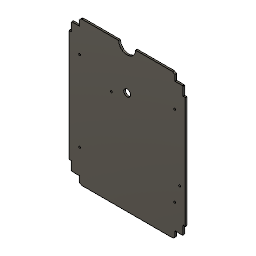
baseplate v1_wire_hole (Autodesk Fusion 360 design; units mm, degrees)
Autodesk Fusion 360 part; units mm, degrees
sketch "Sketch1" plane through (0, 0, 0) normal (0, 0, 1) x (1, 0, 0)
  line L0 (100, 125) -> (-100, 125)
  line L1 (-100, 125) -> (-100, -125)
  line L2 (-100, -125) -> (100, -125)
  line L3 (100, -125) -> (100, 125)
  line L4 (100, 125) -> (-100, -125) construction
  line L5 (-100, 125) -> (100, -125) construction
  line L6 (-100, 125) -> (100, 125)
  line L7 (100, 125) -> (100, 129)
  line L8 (100, 129) -> (-100, 129)
  line L9 (-100, 129) -> (-100, 125)
  line L10 (-100, -125) -> (100, -125)
  line L11 (100, -125) -> (100, -129)
  line L12 (100, -129) -> (-100, -129)
  line L13 (-100, -129) -> (-100, -125)
  line L14 (100, 125) -> (104, 125)
  line L15 (104, 125) -> (104, -125)
  line L16 (104, -125) -> (100, -125)
  line L17 (100, -125) -> (100, 125)
  line L18 (-100, 125) -> (-104, 125)
  line L19 (-104, 125) -> (-104, -125)
  line L20 (-104, -125) -> (-100, -125)
  line L21 (-100, -125) -> (-100, 125)
  line L22 (-80, -53.8) -> (-80, 2.2) construction
  circle A0 centre (-80, -53.8) radius 1.65 construction
  circle A1 centre (-80, 2.2) radius 1.65 construction
  line L23 (-61.0622, -1) -> (-98.9378, -1) construction
  line L24 (-98.9378, -1) -> (-98.9378, -50.6) construction
  line L25 (-98.9378, -50.6) -> (-61.0622, -50.6) construction
  line L26 (-61.0622, -50.6) -> (-61.0622, -1) construction
  line L27 (-61.0622, -1) -> (-98.9378, -50.6) construction
  line L28 (-98.9378, -1) -> (-61.0622, -50.6) construction
  line L29 (-30.5, 49.5) -> (98.5, 49.5) construction
  line L30 (98.5, 49.5) -> (98.5, -47.5) construction
  line L31 (98.5, -47.5) -> (-30.5, -47.5) construction
  line L32 (-30.5, -47.5) -> (-30.5, 49.5) construction
  circle A2 centre (-28, 43) radius 1.65
  circle A3 centre (94, -42) radius 1.65
  line L33 (-100, 125) -> (-85.5, 125)
  line L34 (-85.5, 125) -> (-85.5, 116)
  line L35 (-85.5, 116) -> (-100, 116)
  line L36 (-100, 116) -> (-100, 125)
  line L37 (100, 125) -> (85.5, 125)
  line L38 (85.5, 125) -> (85.5, 116)
  line L39 (85.5, 116) -> (100, 116)
  line L40 (100, 116) -> (100, 125)
  line L41 (-100, -125) -> (-85.5, -125)
  line L42 (-85.5, -125) -> (-85.5, -116)
  line L43 (-85.5, -116) -> (-100, -116)
  line L44 (-100, -116) -> (-100, -125)
  line L45 (100, -125) -> (85.5, -125)
  line L46 (85.5, -125) -> (85.5, -116)
  line L47 (85.5, -116) -> (100, -116)
  line L48 (100, -116) -> (100, -125)
  line L49 (-100, 100) -> (-104, 100)
  line L50 (100, 100) -> (104, 100)
  line L51 (-100, -100) -> (-104, -100)
  line L52 (100, -100) -> (104, -100)
  line L53 (-85.5, 125) -> (-85.5, 129)
  line L54 (85.5, 125) -> (85.5, 129)
  line L55 (-85.5, -125) -> (-85.5, -129)
  line L56 (85.5, -125) -> (85.5, -129)
  line L57 (-115, -140) -> (-75, -140) construction
  line L58 (-75, -140) -> (-75, -87) construction
  line L59 (-75, -87) -> (-115, -87) construction
  line L60 (-115, -87) -> (-115, -140) construction
  line L61 (-63.3606, -140) -> (-21.3606, -140) construction
  line L62 (-21.3606, -140) -> (-21.3606, -53.8) construction
  line L63 (-21.3606, -53.8) -> (-63.3606, -53.8) construction
  line L64 (-63.3606, -53.8) -> (-63.3606, -140) construction
  line L65 (-100, 0) -> (-118.2487, 0) construction
  circle A4 centre (0, 0) radius 152.5
  circle A5 centre (-85, -72) radius 1.65
  line L66 (-85, -72) -> (85, -72) construction
  line L67 (85, -72) -> (85, 72) construction
  line L68 (85, 72) -> (-85, 72) construction
  line L69 (-85, 72) -> (-85, -72) construction
  circle A6 centre (85, 72) radius 1.65
  circle A7 centre (85, -72) radius 1.65
  circle A8 centre (-85, 72) radius 1.65
  point P0 (-80, -25.8)
  dimension "d1" = 200
  dimension "d2" = 250
  dimension "d3" = 4
  dimension "d4" = 4
  dimension "d5" = 4
  dimension "d6" = 4
  dimension "d7" = 20
  dimension "d8" = 56
  dimension "d10" = 3.3
  dimension "d11" = 37.8755
  dimension "d12" = 49.6
  dimension "d13" = 2.5
  dimension "d14" = 6.5
  dimension "d15" = 3.3
  dimension "d16" = 5.5
  dimension "d17" = 4.5
  dimension "d18" = 129
  dimension "d19" = 97
  dimension "d20" = 1.5
  dimension "d21" = 14.5
  dimension "d22" = 9
  dimension "d23" = 14.5
  dimension "d24" = 9
  dimension "d25" = 14.5
  dimension "d26" = 14.5
  dimension "d27" = 9
  dimension "d28" = 9
  dimension "d29" = 25
  dimension "d30" = 25
  dimension "d31" = 25
  dimension "d32" = 25
  dimension "d33" = 40
  dimension "d34" = 53
  dimension "d35" = 15
  dimension "d36" = 15
  dimension "d37" = 3.3
  dimension "d38" = 86.2
  dimension "d39" = 42
  dimension "d40" = 1
  dimension "d50" = 305
  dimension "d51" = 3.3
  dimension "d52" = 15
  dimension "d53" = 15
  dimension "d54" = 15
  dimension "d55" = 53
  dimension "d56" = 53
  dimension "d57" = 170
  dimension "d58" = 144
  dimension "d60" = 47.5
  dimension "d61" = 49.5
  constraint horizontal L0
  constraint perpendicular L0 L1
  constraint parallel L0 L2
  constraint parallel L1 L3
  constraint coincident L4 A4.centre
  constraint coincident L5 A4.centre
  constraint coincident A4.centre origin
  constraint horizontal L6
  constraint vertical L7
  constraint horizontal L8
  constraint vertical L9
  constraint horizontal L10
  constraint vertical L11
  constraint horizontal L12
  constraint vertical L13
  constraint horizontal L14
  constraint vertical L15
  constraint horizontal L16
  constraint vertical L17
  constraint horizontal L18
  constraint vertical L19
  constraint horizontal L20
  constraint vertical L21
  constraint coincident L22.start A0.centre
  constraint coincident L22.end A1.centre
  constraint equal A0 A1
  constraint horizontal L23
  constraint perpendicular L23 L24
  constraint parallel L23 L25
  constraint parallel L24 L26
  constraint coincident L27 P0
  constraint coincident L28 P0
  constraint midpoint L22 P0
  constraint collinear L2 L20
  constraint collinear L11 L17
  constraint collinear L7 L17
  constraint horizontal L29
  constraint vertical L30
  constraint horizontal L31
  constraint vertical L32
  constraint equal A2 A3
  constraint horizontal L33
  constraint vertical L34
  constraint horizontal L35
  constraint vertical L36
  constraint horizontal L37
  constraint vertical L38
  constraint horizontal L39
  constraint vertical L40
  constraint horizontal L41
  constraint vertical L42
  constraint horizontal L43
  constraint vertical L44
  constraint horizontal L45
  constraint vertical L46
  constraint horizontal L47
  constraint vertical L48
  constraint coincident L1 L49.start
  constraint coincident L19 L49.end
  constraint perpendicular L19 L49
  constraint coincident L3 L50.start
  constraint coincident L15 L50.end
  constraint perpendicular L15 L50
  constraint coincident L21 L51.start
  constraint coincident L19 L51.end
  constraint perpendicular L19 L51
  constraint coincident L17 L52.start
  constraint coincident L15 L52.end
  constraint perpendicular L15 L52
  constraint coincident L8 L53.end
  constraint perpendicular L8 L53
  constraint coincident L8 L54.end
  constraint perpendicular L8 L54
  constraint coincident L12 L55.end
  constraint perpendicular L12 L55
  constraint coincident L12 L56.end
  constraint perpendicular L12 L56
  constraint horizontal L57
  constraint vertical L58
  constraint horizontal L59
  constraint vertical L60
  constraint horizontal L61
  constraint vertical L62
  constraint horizontal L63
  constraint vertical L64
  constraint vertical L22
  constraint midpoint L21 L65.start
  constraint perpendicular L19 L65
  constraint collinear L57 L61
  constraint horizontal L66
  constraint vertical L67
  constraint horizontal L68
  constraint vertical L69
  constraint coincident A5.centre L66.start
  constraint coincident L67.end L68.start
  constraint coincident L66.end L67.start
  constraint coincident L68.end L69.start
  constraint equal A6 A8
  constraint equal A5 A7
  constraint equal A6 A7
  measures "d1" distance of L0.start L0.end
  measures "d2" distance of L0.start L2.end
  measures "d3" distance of L0 L8
  measures "d4" distance of L2.end L11.end
  measures "d5" distance of L0.start L14.end
  measures "d6" distance of L0.end L18.end
  measures "d7" distance of L1 L22.start
  measures "d8" distance of L22.start L22.end
  measures "d10" diameter of A1
  measures "d11" distance of L23.start L23.end
  measures "d12" distance of L23.start L25.end
  measures "d13" distance of L32 A2.centre
  measures "d14" distance of L29 A2.centre
  measures "d15" diameter of A2
  measures "d16" distance of L31 A3.centre
  measures "d17" distance of L30 A3.centre
  measures "d18" distance of L29.start L29.end
  measures "d19" distance of L29.end L30.end
  measures "d20" distance of L17 L30
  measures "d21" distance of L34.end L35.end
  measures "d22" distance of L33.end L34.end
  measures "d23" distance of L38.end L39.end
  measures "d24" distance of L37.end L38.end
  measures "d25" distance of L42.end L43.end
  measures "d26" distance of L46.end L47.end
  measures "d27" distance of L41.end L42.end
  measures "d28" distance of L45.end L46.end
  measures "d29" distance of L20 L51
  measures "d30" distance of L18 L49
  measures "d31" distance of L14 L50
  measures "d32" distance of L10 L52
  measures "d33" distance of L57.start L57.end
  measures "d34" distance of L57.start L59.end
  measures "d35" distance of L10 L57
  measures "d36" distance of L21 L60
  measures "d37" diameter of A3
  measures "d38" distance of L61.end L62.end
  measures "d39" distance of L61.start L61.end
  measures "d40" distance of L23 L65
  measures "d50" diameter of A4
  measures "d51" diameter of A5
  measures "d52" distance of L1 A5.centre
  measures "d53" distance of L59 A5.centre
  measures "d54" distance of L17 L67
  measures "d55" distance of L10 L66
  measures "d56" distance of L6 L68
  measures "d57" distance of L67.end L68.end
  measures "d58" distance of L66.end L67.end
  measures "d60" distance of L31 L65
  measures "d61" distance of L29 L65
extrude "Extrude1" add sketch "Sketch1" along normal blind 3 contours L0 L1 L2 L3 L6 L10 L17 L21 L34 L35 L38 L39 L42 L43 L46 L47 A4 | L0 L6 L8 L53 L54 A4 | L3 L15 L17 L50 L52 | L1 L19 L21 L49 L51 | L2 L10 L12 L55 L56 A4
hole "Hole1" at (0, 129, 0) direction (0, 0, 1) diameter 30 depth 10 tip angle 118
hole "Hole2" at (0.013, 55.0023, 0) direction (0, 0, 1) diameter 12 depth 10 tip angle 118
fillet "Fillet1" [suppressed]
fillet "Fillet2" [suppressed]
chamfer "Chamfer1" [suppressed]
fillet "Fillet3" [suppressed]
equation "d4 = d3"
equation "d5 = d3"
equation "d6 = d3"
equation "d23 = d21"
equation "d24 = d22"
equation "d25 = d21"
equation "d26 = d25"
equation "d27 = d22"
equation "d28 = d24"
equation "d30 = d29"
equation "d31 = d29"
equation "d32 = d29"
equation "d36 = d35"
equation "d60 = d19 / 2 - 1 mm"
